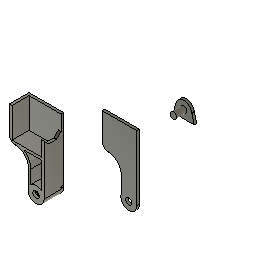
YodaHeatBot_telo (Autodesk Fusion 360 design; units mm, degrees)
Autodesk Fusion 360 part; units mm, degrees
sketch "Sketch1" plane through (0, 0, 0) normal (0, 1, 0) x (1, 0, 0)
  circle A0 centre (25, -25) radius 2.5
  circle A1 centre (25, -25) radius 1.5
  line L0 (25, -11) -> (25, -66.0109) construction
  line L1 (11.5, -20) -> (38.5, -20)
  line L2 (38.5, -20) -> (38.5, -62)
  line L3 (38.5, -62) -> (11.5, -62)
  line L4 (11.5, -62) -> (11.5, -20)
  circle A2 centre (25, -25) radius 5
  circle A3 centre (32.4, -26.1) radius 6
  line L5 (57.6, -57.9991) -> (59.6, -57.9991)
  line L6 (59.6, -57.9991) -> (59.6, -5.9991)
  line L7 (59.6, -5.9991) -> (57.6, -5.9991)
  line L8 (57.6, -39.4991) -> (57.6, -57.9991)
  line L9 (57.6, -3.9991) -> (84.1, -3.9991)
  line L10 (84.1, -3.9991) -> (84.1, -5.9991)
  line L11 (84.1, -5.9991) -> (57.6, -5.9991)
  line L12 (57.6, -5.9991) -> (57.6, -3.9991)
  line L13 (82.1, -57.9991) -> (84.1, -57.9991)
  line L14 (84.1, -57.9991) -> (84.1, -5.9991)
  line L15 (84.1, -5.9991) -> (82.1, -5.9991)
  line L16 (82.1, -5.9991) -> (82.1, -57.9991)
  line L17 (57.6, -59.9991) -> (84.1, -59.9991)
  line L18 (84.1, -59.9991) -> (84.1, -47.9991)
  line L19 (84.1, -57.9991) -> (57.6, -57.9991)
  line L20 (57.6, -57.9991) -> (57.6, -59.9991)
  circle A4 centre (78, -10.0991) radius 6.1
  circle A5 centre (78, -10.0991) radius 2.5
  circle A6 centre (78, -10.0991) radius 1.5
  circle A7 centre (78, -10.0991) radius 2.4
  line L21 (59.6, -36.9991) -> (61.9765, -36.9991)
  line L22 (82.1, -36.9991) -> (82.1, -34.9991)
  line L23 (62.1072, -34.9991) -> (59.6, -34.9991)
  line L24 (59.6, -34.9991) -> (59.6, -36.9991)
  line L25 (82.1, -57.9991) -> (82.1, -59.9991)
  line L26 (59.6, -57.9991) -> (59.6, -59.9991)
  line L27 (70, -3.7991) -> (86, -3.7991)
  line L28 (70, -3.7991) -> (72.1072, -11.6756)
  line L29 (86, -3.7991) -> (83.8928, -11.6756)
  line L30 (82.1, -8.8595) -> (79.8653, -5.9991)
  line L31 (72.1072, -11.6756) -> (72.1072, -24.9991)
  line L32 (82.1, -34.9991) -> (59.6, -34.9991)
  line L33 (62.1, -34.9991) -> (82.1, -34.9991)
  arc A8 (62.1, -34.9991) -> (57.6, -39.4991) centre (62.1, -39.4991) ccw
  arc A9 (62.1072, -34.9991) -> (72.1072, -24.9991) centre (62.1072, -24.9991) ccw
  line L34 (73.9765, -14.684) -> (73.9765, -24.9991)
  arc A10 (61.9765, -36.9991) -> (73.9765, -24.9991) centre (61.9765, -24.9991) ccw
  line L35 (61.9765, -36.9991) -> (82.1, -36.9991)
  point P0 (57.6, -36.9991)
  point P1 (57.6, -34.9991)
  point P2 (82.1, -34.9991)
  dimension "d1" = 5
  dimension "d2" = 3
  dimension "d3" = 27
  dimension "d4" = 42
  dimension "d5" = 6.1
  dimension "d6" = 6.1
  dimension "d7" = 2
  dimension "d8" = 2
  dimension "d9" = 2
  dimension "d10" = 2
  dimension "d12" = 52
  dimension "d13" = 52
  dimension "d14" = 22.5
  dimension "d16" = 26.5
  dimension "d17" = 26.5
  dimension "d18" = 6.1
  dimension "d19" = 5
  dimension "d20" = 3
  dimension "d21" = 4.8
  dimension "d22" = 2
  dimension "d41" = 0.2
  dimension "d42" = 8
  dimension "d43" = 8
  dimension "d50" = 23
  dimension "d55" = 4.5
  dimension "d56" = 10
  dimension "d57" = 12
  constraint concentric A0 A1
  constraint vertical L0
  constraint horizontal L1
  constraint vertical L2
  constraint horizontal L3
  constraint vertical L4
  constraint concentric A1 A2
  constraint horizontal L5
  constraint vertical L6
  constraint horizontal L7
  constraint vertical L8
  constraint horizontal L9
  constraint vertical L10
  constraint horizontal L11
  constraint vertical L12
  constraint horizontal L13
  constraint vertical L14
  constraint horizontal L15
  constraint vertical L16
  constraint horizontal L17
  constraint vertical L18
  constraint horizontal L19
  constraint vertical L20
  constraint coincident L7.end L11.end
  constraint coincident L5.start L8.end
  constraint tangent L14 A4
  constraint tangent L9 A4
  constraint concentric A4 A5
  constraint concentric A5 A6
  constraint concentric A5 A7
  constraint horizontal L21
  constraint vertical L22
  constraint horizontal L23
  constraint vertical L24
  constraint coincident L16 P2
  constraint coincident L6 L21.start
  constraint coincident L17 L25.end
  constraint perpendicular L17 L25
  constraint coincident L17 L26.end
  constraint perpendicular L17 L26
  constraint horizontal L27
  constraint coincident A4 L28.end
  constraint tangent A4 L28
  constraint coincident A4 L29.end
  constraint tangent A4 L29
  constraint coincident L16 L30.start
  constraint coincident L11 L30.end
  constraint coincident L19 L13.start
  constraint coincident L8 P0
  constraint coincident L8 P1
  constraint coincident L23 P2
  constraint perpendicular L21 L31
  constraint coincident P2 L22.end
  constraint perpendicular L31 L33
  constraint coincident L7.end L8
  constraint tangent L33 A8
  constraint tangent L8 A8
  constraint coincident P2 L23
  constraint tangent L23 A9
  constraint tangent L31 A9
  constraint coincident A4 L34.start
  constraint perpendicular L21 L34
  constraint coincident L22.start L21
  constraint tangent L34 A10
  constraint tangent L21 A10
  measures "d1" diameter of A0
  measures "d2" diameter of A1
  measures "d3" distance of L1.start L1.end
  measures "d4" distance of L1.start L3.end
  measures "d5" distance of L2 A3.centre
  measures "d6" distance of L1 A3.centre
  measures "d7" distance of L17.end L13.end
  measures "d8" distance of L5.start L5.end
  measures "d9" distance of L13.start L13.end
  measures "d10" distance of L9.start L7.end
  measures "d12" distance of L5.end L6.end
  measures "d13" distance of L13.end L10.end
  measures "d14" distance of L6 L16
  measures "d16" distance of L17.start L17.end
  measures "d17" distance of L9.start L9.end
  measures "d18" radius of A4
  measures "d19" diameter of A5
  measures "d20" diameter of A6
  measures "d21" diameter of A7
  measures "d22" distance of L21 L23
  measures "d41" distance of L9 L27
  measures "d42" horizontal distance of A4.centre L27.start
  measures "d43" horizontal distance of A4.centre L27.end
  measures "d50" distance of L17 L21
  measures "d55" radius of A8
  measures "d56" radius of A9
  measures "d57" radius of A10
extrude "Extrude1" add sketch "Sketch1" along normal blind 2 contours L5 L6 L8 L19 L24 A8 | L5 L17 L19 L20 L26 | L6 L16 L19 L21 L35 | L17 L19 L25 L26 | L6 L21 L23 L24 L32 L33 A8 A10 | L13 L14 L16 L18 L19 A4 L22 L29 | L13 L17 L18 L19 L25 | L16 L22 L32 L33 A10 L35 | L16 A4 L32 L33 L34 A10 | A4 L31 L32 L33 A9 L34 A10 | L11 L16 A4 L30 | L11 L15 L16 A4 | L11 L16 L30 | L11 L15 A4 makes body 1
extrude "Extrude2" add sketch "Sketch1" against normal blind 13 contours L5 L6 L8 L19 L24 A8 | L5 L17 L19 L20 L26 | L6 L21 L23 L24 L32 L33 A8 A10 | L13 L14 L16 L18 L19 A4 L22 L29 | L13 L17 L18 L19 L25 | L16 L22 L32 L33 A10 L35 | A4 L31 L32 L33 A9 L34 A10 | L14 A4 L29 | L11 L16 A4 L30 | L11 L15 L16 A4 | L11 L16 L30 | L11 L15 A4 bodies 1
extrude "Extrude3" add sketch "Sketch1" against normal blind 2 from surface at 20 separate body contours L5 L6 L8 L19 L24 A8 | L5 L17 L19 L20 L26 | L6 L16 L19 L21 L35 | L17 L19 L25 L26 | L6 L21 L23 L24 L32 L33 A8 A10 | L13 L14 L16 L18 L19 A4 L22 L29 | L13 L17 L18 L19 L25 | L16 L22 L32 L33 A10 L35 | L16 A4 L32 L33 L34 A10 | A4 L31 L32 L33 A9 L34 A10 | L14 A4 L29 | L11 L16 A4 L30 | L11 L15 L16 A4 | L11 L16 L30 | L11 L15 A4 | A5 makes body 2
extrude "Extrude4" cut sketch "Sketch1" against normal blind 3 from surface at 18 contours A5 | A6 | A7 bodies 2
sketch "Sketch2" plane through (84.1, 0, 0) normal (1, 0, 0) x (0, 1, 0)
  line L0 (-13, 10.0991) -> (0, 10.0991)
  line L1 (2, 59.9991) -> (-13, 59.9991)
  line L2 (-13, 59.9991) -> (-13, 10.0991)
  line L3 (0, 62) -> (0, 20)
  line L4 (-13, 44.9991) -> (0, 44.9991)
  line L5 (-13, 59.9991) -> (-13, 36.9991)
  line L6 (-13, 48.4991) -> (-9.5, 44.9991)
  line L7 (-13, 48.4991) -> (-8.0503, 48.4991) construction
  line L8 (0, 48.4806) -> (-3.4815, 44.9991)
  line L9 (0, 10.0991) -> (0, 10.901)
  line L10 (0, 10.901) -> (2, 10.901)
  line L11 (2, 10.901) -> (2, 59.9991)
  point P0 (-13, 36.9991)
  dimension "d38" = 15
  dimension "d54" = 45
  constraint horizontal L4
  constraint coincident L2 L4.start
  constraint coincident L3 L4.end
  constraint horizontal L7
  constraint midpoint L5 L6.start
  constraint coincident L4 L6.end
  constraint coincident L3 L8.start
  constraint coincident L4 L8.end
  constraint perpendicular L6 L8
  measures "d38" distance of L1 L4
  measures "d54" angle of L6 L7
extrude "Extrude6" cut sketch "Sketch2" against normal blind 5 contours L1 L2 L3 L4 L5 L6 L8 bodies 1
move_body "Move1" bodies 2 to x (1, 0, 0) y (0, 1, 0) z (0, 0, 1) at (40, 0, 0)
extrude "Extrude7" add sketch "Sketch1" along normal blind 2 from surface at 100 separate body contours L9 L10 L14 L27 L28 L29 | L11 L16 A4 L30 | L11 L15 L16 A4 | L9 L11 A4 L28 | L11 A4 L28 | L11 L14 L15 A4 | L11 L16 L30 | L11 L15 A4 | L9 L10 L11 L15 A4 | A5 | A6 | A7 makes body 3
extrude "Extrude8" add sketch "Sketch1" against normal blind 8 from surface at 100 contours A6 | A7 bodies 3
extrude "Extrude9" add sketch "Sketch1" along normal blind 4 from surface at -11 contours A5 | A7 bodies 1
